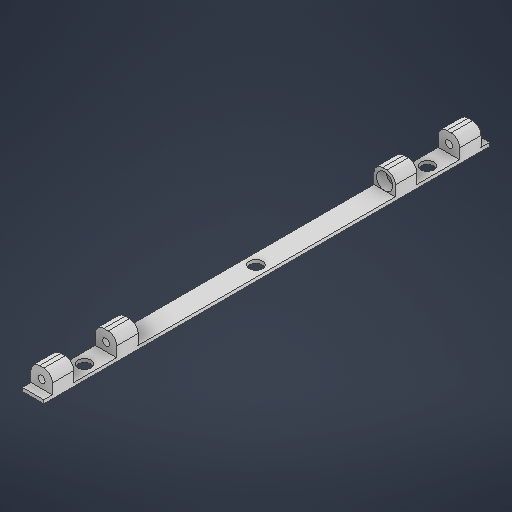
# Autodesk Inventor part: zawias
Saved by Autodesk Inventor 2026.2 (Build 302298010, 298A)
## iProperties
Created: 2026-05-11
Part Number: zawias
Material: Generic
Document SubType Name: Modeling
Designer: karol
Density: 1 g/cm^3
Appearance: Default
Author: karol
Autodesk Inventor part; units mm, degrees
ref_plane "YZ Plane" through (0, 0, 0) normal (1, 0, 0) x (0, 1, 0)
ref_plane "XZ Plane" through (0, 0, 0) normal (0, 1, 0) x (-1, 0, 0)
ref_plane "XY Plane" through (0, 0, 0) normal (0, 0, 1) x (1, 0, 0)
derived "base.ipt"
sketch "Szkic16" plane through (0, 2, 0) normal (0, 1, 0) x (1, 0, 0)
  line L0 (0, -75) -> (0, -40)
  line L1 (0, -75) -> (0, 75)
  line L2 (0, -40) -> (0, 0)
  line L3 (0, -40) -> (0, 0)
  line L4 (0, 0) -> (0, 40)
  line L5 (0, 40) -> (0, 75)
  line L6 (0, -40) -> (0, -30)
  line L7 (0, -30) -> (0, -50)
  line L8 (0, -50) -> (-5, -50)
  line L9 (0, -32) -> (0, -50)
  line L10 (0, 0) -> (0, 10)
  line L11 (0, 10) -> (0, -10)
  line L12 (0, 40) -> (0, 50)
  line L13 (0, 50) -> (0, 30)
  line L14 (0, 30) -> (-5, 30)
  line L15 (0, 46) -> (0, 30)
  line L16 (0, -6) -> (0, 10)
  line L17 (0, -50) -> (-5, -50)
  line L18 (-5, -50) -> (-5, -45)
  line L19 (-5, -45) -> (0, -45)
  line L20 (0, -45) -> (0, -50)
  line L21 (0, -30) -> (-5, -30)
  line L22 (-5, -30) -> (-5, -35)
  line L23 (-5, -35) -> (0, -35)
  line L24 (0, -35) -> (0, -30)
  line L25 (-5, -35) -> (0, -35)
  line L26 (0, -35) -> (0, -45)
  line L27 (0, -45) -> (-5, -45)
  line L28 (-5, -45) -> (-5, -35)
  line L29 (0, -10) -> (-5, -10)
  line L30 (-5, -10) -> (-5, -5)
  line L31 (-5, -5) -> (0, -5)
  line L32 (0, -5) -> (0, -10)
  line L33 (0, 10) -> (-5, 10)
  line L34 (-5, 10) -> (-5, 5)
  line L35 (-5, 5) -> (0, 5)
  line L36 (0, 5) -> (0, 10)
  line L37 (-5, 5) -> (0, 5)
  line L38 (0, 5) -> (0, -5)
  line L39 (0, -5) -> (-5, -5)
  line L40 (-5, -5) -> (-5, 5)
  line L41 (0, 50) -> (-5, 50)
  line L42 (-5, 50) -> (-5, 45)
  line L43 (-5, 45) -> (0, 45)
  line L44 (0, 45) -> (0, 50)
  line L45 (0, 30) -> (-5, 30)
  line L46 (-5, 30) -> (-5, 35)
  line L47 (-5, 35) -> (0, 35)
  line L48 (0, 35) -> (0, 30)
  line L49 (-5, 35) -> (0, 35)
  line L50 (0, 35) -> (0, 45)
  line L51 (0, 45) -> (-5, 45)
  line L52 (-5, 45) -> (-5, 35)
  line L53 (-5, -50) -> (0, -50)
  line L54 (0, -50) -> (0, -52)
  line L55 (0, -52) -> (-5, -52)
  line L56 (-5, -52) -> (-5, -50)
  line L57 (-5, -30) -> (0, -30)
  line L58 (0, -30) -> (0, -28)
  line L59 (0, -28) -> (-5, -28)
  line L60 (-5, -28) -> (-5, -30)
  line L61 (-5, 10) -> (0, 10)
  line L62 (0, 10) -> (0, 12)
  line L63 (0, 12) -> (-5, 12)
  line L64 (-5, 12) -> (-5, 10)
  line L65 (-5, -10) -> (0, -10)
  line L66 (0, -10) -> (0, -12)
  line L67 (0, -12) -> (-5, -12)
  line L68 (-5, -12) -> (-5, -10)
  line L69 (-5, 50) -> (0, 50)
  line L70 (0, 50) -> (0, 52)
  line L71 (0, 52) -> (-5, 52)
  line L72 (-5, 52) -> (-5, 50)
  line L73 (-5, 30) -> (0, 30)
  line L74 (0, 30) -> (0, 28)
  line L75 (0, 28) -> (-5, 28)
  line L76 (-5, 28) -> (-5, 30)
  line L77 (-5, -28) -> (0, -28)
  line L78 (0, -28) -> (0, -12)
  line L79 (0, -12) -> (-5, -12)
  line L80 (-5, -12) -> (-5, -28)
  line L81 (-5, 12) -> (0, 12)
  line L82 (0, 12) -> (0, 28)
  line L83 (0, 28) -> (-5, 28)
  line L84 (-5, 28) -> (-5, 12)
  point P0 (0, 5)
  point P1 (0, -10)
  point P2 (0, -5)
  point P3 (0, -35)
  constraints: 170 end point
extrude "Extrusion10" add sketch "Szkic16" along normal blind 4 contours L8 L18 L19 L0 | L23 L22 L21 L1 | L46 L47 L1 L14 | L42 L41 L1 L43
extrude "Extrusion11" add sketch "Szkic16" against normal blind 1
sketch "Sketch10" plane through (-5, 2, 10) normal (0, 1, 0) x (1, 0, 0)
  line L0 (5, -42) -> (5, -40) projected
  line L1 (0, 62) -> (0, 60) projected
  line L2 (0, 62) -> (0, 60) projected
  line L3 (5, -20) -> (0, -20) projected
  line L4 (5, -42) -> (5, -40) projected
  line L5 (0, -40) -> (5, -40) projected
  line L6 (0, -40) -> (0, -42) projected
  line L7 (0, -42) -> (5, -42) projected
  line L8 (5, -42) -> (5, -40) projected
  line L9 (5, -35) -> (0, -35) projected
  line L10 (5, -35) -> (5, -25) projected
  line L11 (0, -25) -> (5, -25) projected
  line L12 (0, -25) -> (0, -35) projected
  line L13 (5, 60) -> (0, 60) projected
  line L14 (5, 60) -> (5, 62) projected
  line L15 (5, 62) -> (0, 62) projected
  line L16 (0, 62) -> (0, 60) projected
  line L17 (5, 45) -> (0, 45) projected
  line L18 (5, 45) -> (5, 55) projected
  line L19 (0, 55) -> (5, 55) projected
  line L20 (0, 55) -> (0, 45) projected
  line L21 (0, 40) -> (5, 40) projected
  line L22 (0, 62) -> (0, 60) projected
  line L23 (5, -42) -> (5, -40) projected
  line L24 (5, -42) -> (5, -40) projected
  line L25 (0, 62) -> (0, 60) projected
  line L26 (0, 55) -> (5, 55) projected
  line L27 (0, 55) -> (0, 45) projected
  line L28 (5, 45) -> (0, 45) projected
  line L29 (5, 45) -> (5, 55) projected
  line L30 (5, 60) -> (0, 60) projected
  line L31 (5, 60) -> (5, 62) projected
  line L32 (5, 62) -> (0, 62) projected
  line L33 (0, -25) -> (5, -25) projected
  line L34 (0, -25) -> (0, -35) projected
  line L35 (5, -35) -> (0, -35) projected
  line L36 (5, -35) -> (5, -25) projected
  line L37 (5, -20) -> (0, -20) projected
  line L38 (5, -20) -> (5, 40) projected
  line L39 (0, 40) -> (5, 40) projected
  line L40 (0, 40) -> (0, -20) projected
  line L41 (0, -40) -> (5, -40) projected
  line L42 (0, -40) -> (0, -42) projected
  line L43 (0, -42) -> (5, -42) projected
  line L44 (0, 55) -> (5, 55) projected
  line L45 (0, 55) -> (0, 45) projected
  line L46 (5, 45) -> (0, 45) projected
  line L47 (5, 45) -> (5, 55) projected
  line L48 (5, 60) -> (0, 60) projected
  line L49 (5, 60) -> (5, 62) projected
  line L50 (5, 62) -> (0, 62) projected
  line L51 (0, -25) -> (5, -25) projected
  line L52 (0, -25) -> (0, -35) projected
  line L53 (5, -35) -> (0, -35) projected
  line L54 (5, -35) -> (5, -25) projected
  line L55 (5, -20) -> (0, -20) projected
  line L56 (5, -20) -> (5, 40) projected
  line L57 (0, 40) -> (0, -20) projected
  line L58 (0, -40) -> (5, -40) projected
  line L59 (0, -40) -> (0, -42) projected
  line L60 (0, -42) -> (5, -42) projected
  line L61 (0, 55) -> (5, 55) projected
  line L62 (0, 55) -> (0, 45) projected
  line L63 (5, 45) -> (0, 45) projected
  line L64 (5, 45) -> (5, 55) projected
  line L65 (5, 60) -> (0, 60) projected
  line L66 (5, 60) -> (5, 62) projected
  line L67 (5, 62) -> (0, 62) projected
  line L68 (0, -25) -> (5, -25) projected
  line L69 (0, -25) -> (0, -35) projected
  line L70 (5, -35) -> (0, -35) projected
  line L71 (5, -35) -> (5, -25) projected
  line L72 (5, -20) -> (5, 40) projected
  line L73 (0, 40) -> (5, 40) projected
  line L74 (0, 40) -> (0, -20) projected
  line L75 (0, -40) -> (5, -40) projected
  line L76 (0, -40) -> (0, -42) projected
  line L77 (0, -42) -> (5, -42) projected
  line L78 (0, 55) -> (5, 55) projected
  line L79 (0, 55) -> (0, 45) projected
  line L80 (5, 45) -> (0, 45) projected
  line L81 (5, 45) -> (5, 55) projected
  line L82 (5, 60) -> (0, 60) projected
  line L83 (5, 60) -> (5, 62) projected
  line L84 (5, 62) -> (0, 62) projected
  line L85 (0, -25) -> (5, -25) projected
  line L86 (0, -25) -> (0, -35) projected
  line L87 (5, -35) -> (0, -35) projected
  line L88 (5, -35) -> (5, -25) projected
  line L89 (5, -20) -> (0, -20) projected
  line L90 (5, -20) -> (5, 40) projected
  line L91 (0, 40) -> (5, 40) projected
  line L92 (0, 40) -> (0, -20) projected
  line L93 (0, -40) -> (5, -40) projected
  line L94 (0, -40) -> (0, -42) projected
  line L95 (0, -42) -> (5, -42) projected
  point P0 (5, 10)
extrude "Extrusion12" cut sketch "Sketch10" against normal blind 0.4
sketch "Szkic20" plane through (-5, 6, -30) normal (0, 0, 1) x (1, 0, 0)
  circle A0 centre (2.5, -2.5) radius 1.9
  circle A1 centre (2.5, -2.5) radius 0.8
  line L0 (0, -4) -> (0, 0)
  line L1 (0, 0) -> (5, 0)
  point P0 (5, -6)
  constraints: 4 end point, 2 centre point
extrude "Extrusion13" cut sketch "Szkic20" against normal blind 2.2
extrude "Extrusion14" cut sketch "Szkic20" against normal blind 20 contours A1
sketch "Szkic19" plane through (0, 6, 30) normal (0, 0, -1) x (-1, 0, 0)
  circle A0 centre (2.5, -2.5) radius 1.9
  line L0 (0, 0) -> (0, -5)
  line L1 (0, 0) -> (5, 0)
  circle A1 centre (2.5, -2.5) radius 0.8
  point P0 (0, -6)
  point P1 (2.5, 0)
  constraints: 4 end point, 2 centre point
extrude "Extrusion17" cut sketch "Szkic19" against normal blind 2.2 contours A0 | A1
extrude "Extrusion18" cut sketch "Szkic19" against normal blind 20 contours A1
fillet "Fillet1" radius 2 8 edges at (0, 6, 47.5) (-5, 6, 47.5) (0, 6, 32.5) (-5, 6, 32.5) (0, 6, -32.5) (0, 6, -47.5) (-5, 6, -32.5) (-5, 6, -47.5)
sketch "Sketch11" plane through (-5, 1.6, 10) normal (0, 1, 0) x (1, 0, 0)
  circle A0 centre (2.5, -6.7833) radius 1.55
  circle A1 centre (2.5, 25.8333) radius 1.55
  circle A2 centre (2.5, 50) radius 1.55
  circle A3 centre (2.5, -30) radius 1.55
  line L0 (0.6, -20) -> (4.4, -20) projected
  line L1 (0.6, 20) -> (4.4, 20) projected
  line L2 (5, -35) -> (0, -35) projected
  line L3 (0, -35) -> (0, -25) projected
  line L4 (0, -20) -> (0, 62) projected
  line L5 (0, 60) -> (0, 40) projected
  line L6 (0, 45) -> (0, 55) projected
  line L7 (5, 45) -> (0, 45) projected
  point P0 (5, 10)
  point P1 (2.5, -20)
  point P2 (2.5, 20)
  point P3 (2.5, -35)
  point P4 (0, 0)
  point P5 (0, 20)
  point P6 (0, 50)
  point P7 (2.5, 45)
  dimension "d39" = 3.1
  dimension "d40" = 3.1
  dimension "d41" = 3.1
  dimension "d42" = 3.1
  dimension "d43" = 11.6667
  dimension "d44" = 5.8333
  dimension "d45" = 5
  dimension "d46" = 2.5
  dimension "d47" = 2.5
  dimension "d48" = 2.5
  dimension "d49" = 2.5
  dimension "d50" = 5
  constraints: 4 centre point, 3 midpoint
  measures "d39" diameter of A0
  measures "d40" diameter of A1
  measures "d41" diameter of A2
  measures "d42" diameter of A3
  measures "d43" distance edge to line of A0 L0
  measures "d44" distance from line of L1 A1.centre
  measures "d45" distance of A3.centre point (2.5, -35)
  measures "d46" distance from line of L3 A3.centre
  measures "d47" distance from line of L4 A0.centre
  measures "d48" distance from line of L5 A1.centre
  measures "d49" distance of point (0, 50) A2.centre
  measures "d50" distance of point (2.5, 45) A2.centre
extrude "Extrusion19" cut sketch "Sketch11" against normal blind 0.6 contours A2 | A3
sketch "Sketch12" plane through (-5, 1.6, 10) normal (0, 1, 0) x (1, 0, 0)
  circle A0 centre (2.5, 10) radius 1.55
  line L0 (0, 60) -> (0, 62) projected
  line L1 (5, 5) -> (0, 5) projected
  point P0 (5, 10)
  point P1 (0, 15)
  point P2 (0, 10)
  dimension "d53" = 3.1
  dimension "d54" = 2.5
  dimension "d55" = 5
  constraints: 1 centre point, 1 point on line
  measures "d53" diameter of A0
  measures "d54" distance of point (0, 10) A0.centre
  measures "d55" distance from line of L1 A0.centre
extrude "Extrusion20" cut sketch "Sketch12" against normal blind 0.6
sketch "Szkic13" plane through (-5, 1, 52) normal (0, -1, 0) x (1, 0, 0)
  circle A0 centre (2.5, -52) radius 1.55 projected
  circle A1 centre (2.5, -12) radius 1.55 projected
  circle A2 centre (2.5, -92) radius 1.55 projected
  line L0 (5, 0) -> (0, 0) projected
  line L1 (0, 0) -> (0, -104) projected
  line L2 (0, -104) -> (5, -104) projected
  line L3 (5, -104) -> (5, 0) projected
  point P0 (5, -52)
extrude "Wyciągnięcie proste21" add sketch "Szkic13" along normal blind 0.2
body "Solid2"
